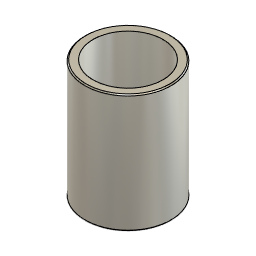
Al. Pipe 16x22mm [(M)SPPS000000057] v2 (Autodesk Fusion 360 design; units mm, degrees)
Autodesk Fusion 360 part; units mm, degrees
sketch "Sketch1" plane through (0, 0, 0) normal (0, 1, 0) x (1, 0, 0)
  circle A0 centre (0, 0) radius 8
  circle A1 centre (0, 0) radius 6.5
  dimension "d1" = 16
  dimension "d2" = 13
  constraint coincident A0.centre A1.centre
  constraint concentric A0 A1
  measures "d1" diameter of A0
  measures "d2" diameter of A1
extrude "Extrude1" add sketch "Sketch1" along normal mid plane 22
chamfer "Chamfer1" distance 0.2 angle 45 2 edges at (-7.4586, 11, 2.8929) (-7.4586, -11, -2.8929)
